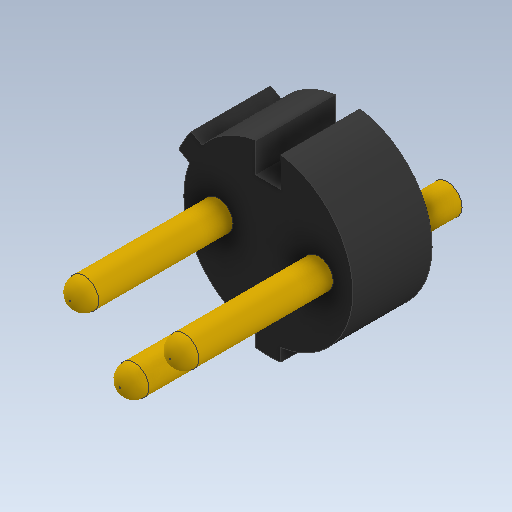
# Autodesk Inventor part: NeutrikXLR
Saved by Autodesk Inventor 2020 (Build 240168000, 168)
## iProperties
Created: 2020-07-05
Part Number: NeutrikXLR
Material: ABS Plastic
Document SubType Name: Modeling
Designer: vmiguel
Density: 1.06 g/cm^3
Appearance: Rubber - Black
Author: vmiguel
Autodesk Inventor part; units mm, degrees
ref_plane "YZ Plane" through (0, 0, 0) normal (1, 0, 0) x (0, 1, 0)
ref_plane "XZ Plane" through (0, 0, 0) normal (0, 1, 0) x (-1, 0, 0)
ref_plane "XY Plane" through (0, 0, 0) normal (0, 0, 1) x (1, 0, 0)
sketch "Sketch1" plane through (0, 0, 0) normal (0, 0, 1) x (1, 0, 0)
  circle A0 centre (0, 0) radius 6.825
  dimension "d0" = 13.65
  constraints: 1 centre point, 1 coincident
  measures "d0" diameter of A0
extrude "Extrusion1" add sketch "Sketch1" along normal blind 6.4
sketch "Sketch2" plane through (0, 0, 6.4) normal (0, 0, 1) x (1, 0, 0)
  circle A0 centre (-4.05, 0) radius 1.2
  circle A1 centre (4.05, 0) radius 1.2
  circle A2 centre (0, -4.05) radius 1.2
  circle A3 centre (0, 0) radius 4.05 construction
  dimension "d3" = 2.4
  dimension "d4" = 2.4
  dimension "d5" = 2.4
  dimension "d6" = 8.1
  constraints: 4 centre point, 3 point on circle, 2 horizontal alignment, 1 coincident, 1 vertical alignment
  measures "d3" diameter of A0
  measures "d4" diameter of A1
  measures "d5" diameter of A2
  measures "d6" diameter of A3
extrude "Extrusion2" add sketch "Sketch2" along normal blind 12
fillet "Fillet1" radius 1.15 3 edges at (-5.25, 0, 18.4) (2.85, 0, 18.4) (-1.2, -4.05, 18.4)
sketch "Sketch3" plane through (0, 0, 0) normal (0, 0, -1) x (-1, 0, 0)
  circle A0 centre (-4.05, 0) radius 1.2 projected
  circle A1 centre (4.05, 0) radius 1.2 projected
  circle A2 centre (0, -4.05) radius 1.2 projected
  point P0 (0, 0)
extrude "Extrusion3" add sketch "Sketch3" along normal blind 4
sketch "Sketch4" plane through (0, 0, 6.4) normal (0, 0, 1) x (1, 0, 0)
  line L0 (-1, 6.825) -> (1, 6.825)
  line L1 (1, 6.825) -> (1, 4.325)
  line L2 (1, 4.325) -> (-1, 4.325)
  line L3 (-1, 4.325) -> (-1, 6.825)
  circle A0 centre (0, 0) radius 6.825 projected
  point P0 (0, 4.325)
  point P1 (0, 6.825)
  point P2 (1, 6.7513)
  point P3 (-1, 6.7513)
  dimension "d12" = 2
  dimension "d13" = 2.5
  constraints: 8 end point, 2 midpoint, 2 parallel, 1 horizontal, 1 perpendicular, 1 vertical alignment, 2 other
  measures "d12" distance of L1.end L2.end
  measures "d13" distance of L0.end L1.end
extrude "Extrusion4" cut sketch "Sketch4" against normal through all contours A0 L1 L2 L3 picked at (0, 5.1583)
sketch "Sketch5" plane through (0, 0, 6.4) normal (0, 0, 1) x (1, 0, 0)
  arc A0 (-1, 6.7513) -> (1, 6.7513) centre (0, 0) ccw projected
  arc A1 (-1.1465, 7.7406) -> (1.1465, 7.7406) centre (0, 0) ccw
  arc A2 (-1, 6.7513) -> (1, 6.7513) centre (0, 0) ccw projected
  line L0 (-1, -6.7513) -> (-1, -7.7608)
  line L1 (1, -6.7513) -> (1, -7.7608)
  dimension "d16" = 1
  dimension "d17" = 1
  dimension "d18" = 1
  constraints: 6 point on circle, 4 end point, 1 centre point, 1 parallel, 1 vertical
  measures "d16" distance from line of L1 point (0, 0)
  measures "d17" distance from line of L0 point (0, 0)
  measures "d18" radial gap between concentric circles of A0 A1
extrude "Extrusion5" add sketch "Sketch5" against normal up to surface (6.4 mm away)
pattern_circular "Circular Pattern1" count 2 over 120 about axis through (0, 0, 0) along (0, 0, -1) of "Extrusion5"
body "Solid1"
